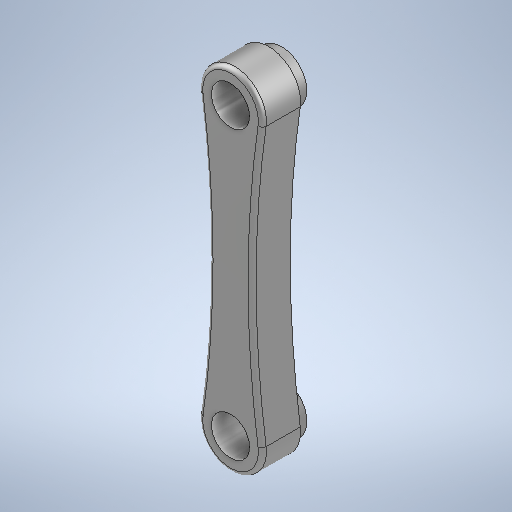
# Autodesk Inventor part: Robot_arm_1
Saved by Autodesk Inventor 2025 (Build 290162010, 162A)
## iProperties
Created: 2024-07-13
Part Number: Robot_arm_1
Material: Generic
Document SubType Name: Modeling
Designer: saees
Density: 1 g/cm^3
Appearance: Anodized - Light Gray
Author: saees
Autodesk Inventor part; units mm, degrees
ref_plane "YZ Plane" through (0, 0, 0) normal (1, 0, 0) x (0, 1, 0)
ref_plane "XZ Plane" through (0, 0, 0) normal (0, 1, 0) x (-1, 0, 0)
ref_plane "XY Plane" through (0, 0, 0) normal (0, 0, 1) x (1, 0, 0)
sketch "Sketch1" plane through (0, 0, 0) normal (0, 0, 1) x (1, 0, 0)
  circle A0 centre (0, 0) radius 50
  circle A1 centre (0, 450) radius 50
  arc A2 (49.4865, 442.8526) -> (49.4865, 7.1474) centre (1557.8354, 225) ccw
  arc A3 (-49.4865, 7.1474) -> (-49.4865, 442.8526) centre (-1557.8354, 225) ccw
  dimension "d0" = 100
  dimension "d1" = 450
  dimension "d2" = 1524
  constraints: 8 point on circle, 4 centre point, 4 tangent, 2 equal radius, 1 coincident, 1 vertical alignment
  measures "d0" diameter of A0
  measures "d1" distance of point (0, 0) A1.centre
  measures "d2" radius of A2
extrude "Extrusion1" add sketch "Sketch1" along normal blind 60
fillet "Fillet1" radius 6.35 4 edges at (-33.8354, 225, 60) (0, -50, 60) (33.8354, 225, 60) (0, 500, 60)
sketch "Sketch2" plane through (0, 0, 0) normal (0, 0, -1) x (-1, 0, 0)
  circle A0 centre (0, 450) radius 40
  circle A1 centre (0, 0) radius 40
  arc A2 (49.4865, 442.8526) -> (49.4865, 7.1474) centre (1557.8354, 225) ccw projected
  arc A3 (49.4865, 442.8526) -> (-49.4865, 442.8526) centre (0, 450) ccw projected
  arc A4 (-49.4865, 7.1474) -> (-49.4865, 442.8526) centre (-1557.8354, 225) ccw projected
  arc A5 (-49.4865, 7.1474) -> (49.4865, 7.1474) centre (0, 0) ccw projected
  dimension "d6" = 80
  constraints: 2 centre point, 2 coincident, 1 equal radius
  measures "d6" diameter of A0
extrude "Extrusion2" add sketch "Sketch2" along normal blind 20 contours A0 | A1
sketch "Sketch3" plane through (0, 0, 60) normal (0, 0, 1) x (1, 0, 0)
  circle A0 centre (0, 0) radius 30
  arc A1 (-43.2017, 6.2397) -> (-43.2017, 443.7603) centre (-1557.8354, 225) ccw projected
  arc A2 (-43.2017, 6.2397) -> (43.2017, 6.2397) centre (0, 0) ccw projected
  arc A3 (43.2017, 443.7603) -> (43.2017, 6.2397) centre (1557.8354, 225) ccw projected
  arc A4 (43.2017, 443.7603) -> (-43.2017, 443.7603) centre (0, 450) ccw projected
  circle A5 centre (0, 450) radius 30
  dimension "d9" = 60
  constraints: 2 centre point, 2 coincident, 1 equal radius
  measures "d9" diameter of A5
extrude "Extrusion3" cut sketch "Sketch3" against normal blind 70 contours A0 | A5
sketch "Sketch4" plane through (0, 450, -10) normal (0, 0, 1) x (1, 0, 0)
  circle A0 centre (0, 0) radius 30 projected
  circle A1 centre (0, -450) radius 30 projected
  circle A2 centre (0, 0) radius 2.5
  circle A3 centre (0, -450) radius 2.5
  dimension "d12" = 5
  constraints: 2 centre point, 2 coincident, 1 equal radius
  measures "d12" diameter of A2
extrude "Extrusion4" cut sketch "Sketch4" against normal through all contours A2 | A3
body "Solid1"
